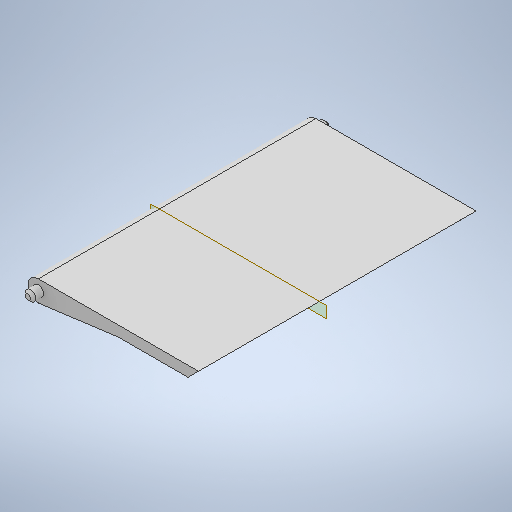
# Autodesk Inventor part: Part7v2
Saved by Autodesk Inventor 2025.2 (Build 292293000, 293)
## iProperties
Created: 2025-06-06
Part Number: Part7v2
Material: Generic
Document SubType Name: Sheet Metal
Designer: ziyuz
Density: 1 g/cm^3
Sheet Metal Rule: Default_mm
Appearance: Default
Author: ziyuz
Autodesk Inventor part; units mm, degrees
ref_plane "YZ Plane" through (0, 0, 0) normal (1, 0, 0) x (0, 1, 0)
ref_plane "XZ Plane" through (0, 0, 0) normal (0, 1, 0) x (-1, 0, 0)
ref_plane "XY Plane" through (0, 0, 0) normal (0, 0, 1) x (1, 0, 0)
sketch "Sketch1" plane through (0, 0, 0) normal (0, 1, 0) x (-1, 0, 0)
  line L0 (0, 0) -> (-30.566, 0)
  line L1 (-30.566, 0) -> (-30.566, -53)
  line L2 (-30.566, -53) -> (0, -53)
  line L3 (0, -53) -> (0, 0)
  dimension "d0" = 30.566
  dimension "d1" = 53
  constraints: 8 end point, 2 parallel, 1 horizontal, 1 perpendicular
  measures "d0" distance of L2.end L1.end
  measures "d1" distance of L1.end L0.end
extrude "Extrusion1" add sketch "Sketch1" along normal blind 2
ref_plane "Work Plane1" through (30.566, 0, -23) normal (0, 0, -1) x (-1, 0, 0)
sketch "Sketch2" plane through (30.566, 0, -23) normal (0, 0, -1) x (-1, 0, 0)
  point P0 (30.566, 0)
sketch "Sketch3" plane through (30.566, 0, -53) normal (0, 0, -1) x (-1, 0, 0)
  circle A0 centre (30.566, 0) radius 1
  circle A1 centre (30.566, 0) radius 2
  line L0 (30.566, -2) -> (15.283, 0)
  line L1 (15.283, 0) -> (28.566, 0)
  line L2 (0, 0) -> (30.566, 0) projected
  dimension "d5" = 2
  dimension "d6" = 4
  constraints: 4 end point, 2 centre point, 2 coincident, 2 point on circle, 1 point on line
  measures "d5" diameter of A0
  measures "d6" diameter of A1
extrude "Extrusion2" add sketch "Sketch3" against normal blind 53 contours A1 L0 | A1 L0 L1 picked at (30.3543, -1.6418)
sketch "Sketch4" plane through (30.566, 0, -53) normal (0, 0, -1) x (-1, 0, 0)
  arc A0 (29.566, 0) -> (30.566, 1) centre (30.566, 0) ccw projected
  circle A1 centre (30.566, 0) radius 1
  point P0 (30.566, 1)
  constraints: 1 coincident, 3 other
extrude "Extrusion3" cut sketch "Sketch4" against normal blind 53
chamfer "Chamfer2" distance 2 angle 45 1 edges at (30.566, 0, -26.5)
sketch "Sketch5" plane through (0, 0, 0) normal (0, 0, 1) x (1, 0, 0)
  circle A0 centre (0, 0) radius 1
  constraints: 1 centre point, 1 coincident
extrude "Extrusion4" add sketch "Sketch5" along normal blind 2 and the other way blind 55
chamfer "Chamfer3" distance 0.5 angle 45 1 edges at (-1, 0, 2)
chamfer "Chamfer4" distance 0.5 angle 45 1 edges at (-1, 0, -55)
equation "\"BendRadius\" = Thickness"
equation "\"BendReliefWidth\" = Thickness"
equation "\"BendReliefDepth\" = 0.5 * Thickness"
equation "\"CornerReliefSize\" = 4 * Thickness"
equation "\"MinimumRemnant\" = 2 * Thickness"
equation "\"TransitionRadius\" = BendRadius"
equation "\"JacobiRadiusSize\" = BendRadius"
equation "\"GapSize\" = Thickness"
equation "\"Thickness\" = 0.5"
body "Solid1"
